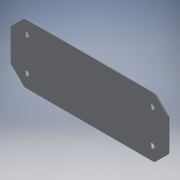
# Autodesk Inventor part: Nameplatedrill
Saved by Autodesk Inventor 2018.3 (Build 223284000, 284)
## iProperties
Created: 2019-08-17
Part Number: Nameplatedrill
Material: Generic
Document SubType Name: Modeling
Designer: Srinity
Density: 1 g/cm^3
Appearance: Default
Author: Srinity
Autodesk Inventor part; units mm, degrees
ref_plane "YZ Plane" through (0, 0, 0) normal (1, 0, 0) x (0, 1, 0)
ref_plane "XZ Plane" through (0, 0, 0) normal (0, 1, 0) x (-1, 0, 0)
ref_plane "XY Plane" through (0, 0, 0) normal (0, 0, 1) x (1, 0, 0)
sketch "Sketch1" plane through (0, 0, 0) normal (0, 0, 1) x (1, 0, 0)
  circle A0 centre (-114.3, -4.6736) radius 2.1 projected
  circle A1 centre (-114.3, -35.1536) radius 2.1 projected
  circle A2 centre (0, -35.1536) radius 2.1 projected
  circle A3 centre (0, -4.6736) radius 2.1 projected
  line L0 (-114.9665, 7.2136) -> (0.6665, 7.2136) projected
  arc A4 (2.8956, 6.2995) -> (0.6665, 7.2136) centre (0.6665, 4.0386) ccw projected
  line L1 (2.8956, 6.2995) -> (13.6591, -4.3125) projected
  arc A5 (14.605, -6.5734) -> (13.6591, -4.3125) centre (11.43, -6.5734) ccw projected
  line L2 (14.605, -6.5734) -> (14.605, -33.2538) projected
  arc A6 (13.6591, -35.5147) -> (14.605, -33.2538) centre (11.43, -33.2538) ccw projected
  line L3 (13.6591, -35.5147) -> (2.8956, -46.1267) projected
  line L4 (0.6665, -47.0408) -> (-114.9665, -47.0408) projected
  arc A7 (0.6665, -47.0408) -> (2.8956, -46.1267) centre (0.6665, -43.8658) ccw projected
  arc A8 (-117.1956, -46.1267) -> (-114.9665, -47.0408) centre (-114.9665, -43.8658) ccw projected
  line L5 (-117.1956, -46.1267) -> (-127.9591, -35.5147) projected
  arc A9 (-128.905, -33.2538) -> (-127.9591, -35.5147) centre (-125.73, -33.2538) ccw projected
  line L6 (-128.905, -33.2538) -> (-128.905, -6.5734) projected
  arc A10 (-127.9591, -4.3125) -> (-128.905, -6.5734) centre (-125.73, -6.5734) ccw projected
  line L7 (-127.9591, -4.3125) -> (-117.1956, 6.2995) projected
  arc A11 (-114.9665, 7.2136) -> (-117.1956, 6.2995) centre (-114.9665, 4.0386) ccw projected
  point P0 (0, 0)
extrude "Extrusion1" add sketch "Sketch1" along normal blind 1
body "Solid1"
